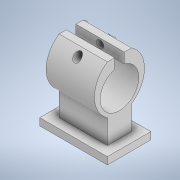
# Autodesk Inventor part: Clamp
Saved by Autodesk Inventor 2021 (Build 250183000, 183)
## iProperties
Created: 2021-05-12
Part Number: Clamp
Material: Generic
Document SubType Name: Modeling
Designer: chick
Density: 1 g/cm^3
Appearance: Default
Author: chick
Autodesk Inventor part; units mm, degrees
ref_plane "YZ Plane" through (0, 0, 0) normal (1, 0, 0) x (0, 1, 0)
ref_plane "XZ Plane" through (0, 0, 0) normal (0, 1, 0) x (-1, 0, 0)
ref_plane "XY Plane" through (0, 0, 0) normal (0, 0, 1) x (1, 0, 0)
sketch "Sketch1" plane through (0, 0, 0) normal (1, 0, 0) x (0, 1, 0)
  line L0 (0, -4.8819) -> (5, -4.8819)
  line L1 (5, -4.8819) -> (0, -4.8819)
  line L2 (0, -4.8819) -> (0, -9.8819)
  line L3 (0, -9.8819) -> (5, -9.8819)
  arc A0 (15, -4.8819) -> (5, -4.8819) centre (10, -8.1985) ccw
  arc A1 (5, -9.8819) -> (15, -9.8819) centre (10, -6.5653) ccw
  line L4 (15, -9.8819) -> (15, -4.8819)
  point P0 (0, 0)
  point P1 (0, -7.3819)
  point P2 (10, -7.3819)
  point P3 (10, -4.8819)
  point P4 (10, -9.8819)
  dimension "d0" = 5
  dimension "d1" = 10
  dimension "d2" = 5
  dimension "d3" = 5
  dimension "d4" = 10
  dimension "d5" = 6
  dimension "d6" = 6
  constraints: 10 end point, 4 point on circle, 2 centre point, 2 vertical, 1 collinear, 1 horizontal, 1 midpoint, 1 perpendicular
  measures "d0" distance of L0.start L2.end
  measures "d1" distance of point (10, -7.382) point (0, -7.382)
  measures "d2" distance of L0.start L0.end
  measures "d3" distance of L2.end L3.end
  measures "d4" distance of L0.end L4.end
  measures "d5" radius of A0
  measures "d6" radius of A1
extrude "Extrusion1" add sketch "Sketch1" along normal blind 10
sketch "Sketch7" plane through (10, 0, 0) normal (1, 0, 0) x (0, 0, -1)
  line L0 (9.8819, 15) -> (4.8819, 15) projected
  line L1 (9.8819, 0) -> (9.8819, 5) projected
  line L2 (4.8819, 0) -> (9.8819, 0) projected
  circle A0 centre (7.3819, 9) radius 4
  point P0 (0, 0)
  point P1 (7.3819, 15)
  point P2 (7.3819, 5)
  point P3 (9.8819, 10.0351)
  dimension "d29" = 2.5
  dimension "d30" = 10
  dimension "d31" = 4
  dimension "d33" = 5
  constraints: 1 coincident, 1 midpoint, 1 vertical alignment, 2 other
  measures "d29" distance from line of point (7.382, 15) L1
  measures "d30" distance from line of L0 L1.end
  measures "d31" distance of point (7.382, 5) point (7.382, 9)
  measures "d33" distance from line of L2 point (7.382, 5)
extrude "Extrusion4" cut sketch "Sketch7" against normal blind 10
sketch "Sketch8" plane through (10, 0, 0) normal (1, 0, 0) x (0, 0, -1)
  line L0 (8.3819, 12.873) -> (8.3819, 15)
  line L1 (9.8819, 15) -> (4.8819, 15) projected
  line L2 (9.8819, 15) -> (4.8819, 15) projected
  line L3 (6.3819, 15) -> (6.3819, 12.873)
  circle A0 centre (7.3819, 9) radius 4 projected
  line L4 (8.3819, 15) -> (6.3819, 15)
  arc A1 (8.3819, 12.873) -> (6.3819, 12.873) centre (7.3819, 9) ccw
  point P0 (0, 0)
  dimension "d36" = 1.5
  dimension "d39" = 1.5
  constraints: 6 end point, 3 point on circle, 2 point on line, 2 vertical, 1 centre point, 1 collinear, 1 concentric
  measures "d36" distance of L0.end L1.start
  measures "d39" distance of L1.end L3.start
extrude "Extrusion5" cut sketch "Sketch8" against normal blind 10 contours A0 L3 L1 L0
sketch "Sketch9" plane through (0, 0, -9.8819) normal (0, 0, -1) x (-1, 0, 0)
  circle A0 centre (-5, 13.9365) radius 0.4
  line L0 (-10, 12.873) -> (0, 12.873) projected
  line L1 (0, 15) -> (-10, 15) projected
  line L2 (-10, 15) -> (-10, 5) projected
  point P0 (0, 0)
  dimension "d42" = 0.8
  dimension "d43" = 1.0635
  dimension "d44" = 2.127
  dimension "d45" = 10
  dimension "d46" = 5
  constraints: 1 centre point
  measures "d42" diameter of A0
  measures "d43" distance from line of L0 A0.centre
  measures "d44" distance between parallel lines of L1 L0
  measures "d45" distance of L1.start L1.end
  measures "d46" distance from line of L2 A0.centre
hole "Hole1" at (5, 13.9365, -9.8819) direction (0, 0, -1) diameter 1.5 end through all both
sketch "Sketch10" plane through (0, 0, -9.8819) normal (0, -1, 0) x (1, 0, 0)
  line L0 (12, -2) -> (12, 7)
  line L1 (12, 7) -> (-2, 7)
  line L2 (0, 7.6834) -> (10, 7.6834) projected
  line L3 (-2, 7) -> (-2, -2)
  line L4 (-2, -2) -> (12, -2)
  line L5 (0, -2.6834) -> (10, -2.6834) projected
  line L6 (0, -2.6834) -> (0, 0) projected
  line L7 (0, 0) -> (10, 0) projected
  line L8 (0, 5) -> (0, 0) projected
  line L9 (0, 5) -> (10, 5) projected
  point P0 (0, 9.8819)
  point P1 (5, 2.5)
  dimension "d54" = 14
  dimension "d56" = 2
  dimension "d57" = 2
  dimension "d58" = 5
  dimension "d59" = 2.5
  dimension "d60" = 2
  dimension "d74" = 9
  constraints: 8 end point, 2 parallel, 1 perpendicular, 1 vertical
  measures "d54" distance of L3.end L0.start
  measures "d56" distance between parallel lines of L3 L6
  measures "d57" distance between parallel lines of L7 L4
  measures "d58" distance from line of L8 point (5, 2.5)
  measures "d59" distance from line of L9 point (5, 2.5)
  measures "d60" distance between parallel lines of L1 L9
  measures "d74" distance of L0.start L0.end
extrude "Extrusion6" add sketch "Sketch10" along normal blind 1.5
sketch "Sketch11" plane through (10, 0, 0) normal (1, 0, 0) x (0, 0, -1)
  point P0 (0, 0)
sketch "Sketch12" plane through (0, -1.5, -9.8819) normal (0, -1, 0) x (1, 0, 0)
  line L0 (-2, 7) -> (-2, -2) projected
  line L1 (12, 7) -> (-2, 7) projected
  circle A0 centre (5, 2.5) radius 2.5
  point P0 (0, 9.8819)
  dimension "d63" = 7
  dimension "d64" = 4.5
  dimension "d65" = 9
  dimension "d66" = 5
  constraints: 1 centre point, 1 coincident
  measures "d63" distance from line of point (5, 2.5) L0
  measures "d64" distance from line of point (5, 2.5) L1
  measures "d65" distance of L0.start L0.end
  measures "d66" diameter of A0
hole "Hole2" at (5, -1.5, -7.3819) direction (0, 1, 0) diameter 5 depth 1.5
equation "\"d2\" = d0"
equation "\"d3\" = d0"
equation "\"d36\" = d37"
equation "\"d43\" = 0.5 * d44"
equation "\"d59\" = 0.5 * d58"
equation "\"d60\" = d57"
equation "\"d64\" = 0.5 * d65"
equation "\"d66\" = hoop_bearing_length"
equation "\"hoop_bearing_length\" = 5"
equation "\"d37\" = 1.5"
body "Solid1"
